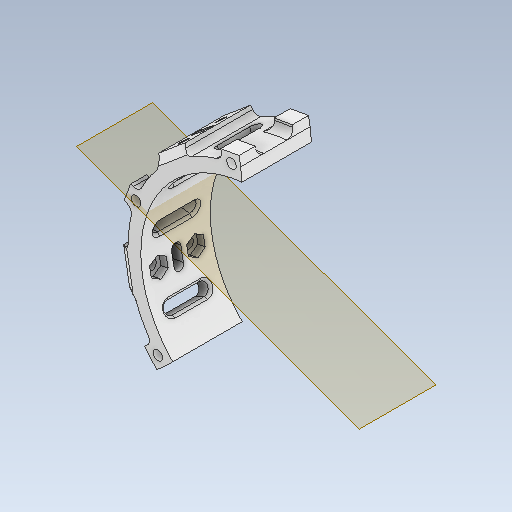
# Autodesk Inventor part: shell_3
Saved by Autodesk Inventor 2020 (Build 240168000, 168)
## iProperties
Created: 2020-07-11
Part Number: shell_3
Material: ABS Plastic
Document SubType Name: Modeling
Designer: psrobotics
Density: 1.06 g/cm^3
Appearance: Smooth - White
Author: psrobotics
Autodesk Inventor part; units mm, degrees
sketch "Sketch1" plane through (0, 0, 0) normal (0, 0, 1) x (1, 0, 0)
  line L0 (52.6477, -39.8597) -> (50.9677, -42.7938) projected
  line L1 (39.9879, -61.9696) -> (50.9677, -42.7938) projected
  circle A0 centre (0, 0) radius 5.9 projected
  circle A1 centre (0, 0) radius 45.5 projected
  circle A2 centre (0, 0) radius 48.5
  circle A3 centre (0, 0) radius 54
  line L2 (0, 0) -> (0, -54)
  line L3 (0, 0) -> (0, 54)
  line L4 (0, 0) -> (-18.4691, -50.7434)
  line L5 (-18.4691, -50.7434) -> (-18.4691, -50.7434)
  line L6 (-26.7139, -51.4672) -> (-12.6185, -56.5975)
  line L7 (-12.6185, -56.5975) -> (-10.2243, -50.0196)
  line L8 (-10.2243, -50.0196) -> (-24.3197, -44.8893)
  line L9 (-24.3197, -44.8893) -> (-26.7139, -51.4672)
  line L10 (-26.7139, -51.4672) -> (-10.2243, -50.0196) construction
  line L11 (-12.6185, -56.5975) -> (-24.3197, -44.8893) construction
  line L12 (-57.9288, -2.5987) -> (-55.3241, -17.3708)
  line L13 (-55.3241, -17.3708) -> (-48.4304, -16.1553)
  line L14 (-48.4304, -16.1553) -> (-51.0352, -1.3832)
  line L15 (-51.0352, -1.3832) -> (-57.9288, -2.5987)
  line L16 (-31.215, 48.8685) -> (-42.7056, 39.2266)
  line L17 (-42.7056, 39.2266) -> (-38.2061, 33.8643)
  line L18 (-38.2061, 33.8643) -> (-26.7154, 43.5062)
  line L19 (-26.7154, 43.5062) -> (-31.215, 48.8685)
  line L20 (26.7139, 51.4672) -> (12.6185, 56.5975)
  line L21 (12.6185, 56.5975) -> (10.2243, 50.0196)
  line L22 (10.2243, 50.0196) -> (24.3197, 44.8893)
  line L23 (24.3197, 44.8893) -> (26.7139, 51.4672)
  line L24 (-10.2243, -50.0196) -> (24.3197, 44.8893)
  point P0 (0, 0)
  point P1 (-9.3407, -47.592)
  point P2 (23.4361, 42.4617)
  point P3 (11.2424, 52.8167)
  point P4 (-28.6288, 45.7864)
  point P5 (-40.1194, 36.1446)
  point P6 (-53.9666, -1.9001)
  point P7 (-51.3618, -16.6722)
  point P8 (-25.3378, -47.6864)
  dimension "d0" = 97
  dimension "d1" = 108
  dimension "d2" = 54
  dimension "d3" = 20
  dimension "d4" = 0
  dimension "d5" = 15
  dimension "d6" = 7
  dimension "d9" = 180
  constraints: 46 end point, 2 centre point, 2 coincident, 2 midpoint, 2 parallel, 2 perpendicular, 2 point on circle, 2 vertical, 1 collinear, 25 other
  measures "d0" diameter of A2
  measures "d1" diameter of A3
  measures "d2" distance of L2.start L4.end
  measures "d3" angle of L2 L4
  measures "d4" distance of L4.end L5.end
  measures "d5" distance of L6.start L6.end
  measures "d6" distance of L7.end L6.end
extrude "Extrusion1" add sketch "Sketch1" against normal blind 30 contours L3 A3 L21 L22 L24 A2 | A2 L4 L8 L9 A3 L13 L14 L15 L17 L18 L19 L3 | A2 L24 L8 L4 | L8 L7 A3 L4 | L4 A3 L9 L8 | L22 L21 A3 L23 | L21 L20 L23 A3 | L19 L18 L17 A3 | A3 L17 L16 L19 | A3 L7 L6 L9 | L15 L14 L13 A3 | A3 L13 L12 L15
sketch "Sketch2" plane through (0, 0, -30) normal (0, 0, -1) x (-1, 0, 0)
  line L0 (57.9288, -2.5987) -> (53.9666, -1.9001) projected
  arc A0 (53.9666, -1.9001) -> (40.1194, 36.1446) centre (0, 0) ccw projected
  line L1 (40.1194, 36.1446) -> (42.7056, 39.2266) projected
  line L2 (42.7056, 39.2266) -> (31.215, 48.8685) projected
  line L3 (31.215, 48.8685) -> (28.6288, 45.7864) projected
  arc A1 (28.6288, 45.7864) -> (-11.2424, 52.8167) centre (0, 0) ccw projected
  line L4 (-11.2424, 52.8167) -> (-12.6185, 56.5975) projected
  line L5 (-12.6185, 56.5975) -> (-26.7139, 51.4672) projected
  line L6 (-26.7139, 51.4672) -> (-23.4361, 42.4617) projected
  arc A2 (9.3407, -47.592) -> (-23.4361, 42.4617) centre (0, 0) ccw projected
  line L7 (9.3407, -47.592) -> (12.6185, -56.5975) projected
  line L8 (12.6185, -56.5975) -> (26.7139, -51.4672) projected
  line L9 (26.7139, -51.4672) -> (25.3378, -47.6864) projected
  arc A3 (25.3378, -47.6864) -> (51.3618, -16.6722) centre (0, 0) ccw projected
  line L10 (51.3618, -16.6722) -> (55.3241, -17.3708) projected
  line L11 (55.3241, -17.3708) -> (57.9288, -2.5987) projected
  line L12 (0, 0) -> (-19.6662, 54.0323)
  line L13 (-26.7139, 51.4672) -> (-12.6185, 56.5975) projected
  line L14 (-16.588, 45.5751) -> (-23.6357, 43.0099)
  line L15 (-23.4361, 42.4617) -> (-26.7139, 51.4672) projected
  point P0 (0, 0)
  constraints: 4 end point, 2 perpendicular, 2 point on line, 1 midpoint, 1 point on circle
extrude "Extrusion2" cut sketch "Sketch2" against normal blind 50 contours A2 L6 L14
ref_plane "Work Plane1" through (7.0477, -2.5652, 0) normal (0.3420201, 0.9396926, 0) x (0.9396926, -0.3420201, 0)
mirror "Mirror1" about plane through (7.0477, -2.5652, 0) normal (0.3420201, 0.9396926, 0) of "Extrusion2"
sketch "Sketch3" plane through (0, 0, 0) normal (0, 0, 1) x (1, 0, 0)
  line L0 (-9.5403, -48.1402) -> (-16.588, -45.5751) projected
  arc A0 (16.588, 45.5751) -> (-16.588, -45.5751) centre (0, 0) ccw projected
  line L1 (16.588, 45.5751) -> (23.6357, 43.0099) projected
  line L2 (23.6357, 43.0099) -> (26.7139, 51.4672) projected
  line L3 (26.7139, 51.4672) -> (12.6185, 56.5975) projected
  line L4 (12.6185, 56.5975) -> (11.2424, 52.8167) projected
  arc A1 (11.2424, 52.8167) -> (-28.6288, 45.7864) centre (0, 0) ccw projected
  line L5 (-28.6288, 45.7864) -> (-31.215, 48.8685) projected
  line L6 (-31.215, 48.8685) -> (-42.7056, 39.2266) projected
  line L7 (-42.7056, 39.2266) -> (-40.1194, 36.1446) projected
  arc A2 (-40.1194, 36.1446) -> (-53.9666, -1.9001) centre (0, 0) ccw projected
  line L8 (-53.9666, -1.9001) -> (-57.9288, -2.5987) projected
  line L9 (-57.9288, -2.5987) -> (-55.3241, -17.3708) projected
  line L10 (-55.3241, -17.3708) -> (-51.3618, -16.6722) projected
  arc A3 (-51.3618, -16.6722) -> (-25.3378, -47.6864) centre (0, 0) ccw projected
  line L11 (-25.3378, -47.6864) -> (-26.7139, -51.4672) projected
  line L12 (-26.7139, -51.4672) -> (-12.6185, -56.5975) projected
  line L13 (-12.6185, -56.5975) -> (-9.5403, -48.1402) projected
  line L14 (-12.6185, -56.5975) -> (-26.7139, -51.4672) projected
  line L15 (-19.6662, -54.0323) -> (-56.6264, -9.9848)
  line L16 (-55.3241, -17.3708) -> (-57.9288, -2.5987) projected
  line L17 (0, 0) -> (-38.1463, -32.0085)
  line L18 (-38.1463, -32.0085) -> (-41.2105, -34.5797)
  line L19 (-41.7035, -40.215) -> (-46.8458, -34.0867)
  line L20 (-46.8458, -34.0867) -> (-40.7175, -28.9444)
  line L21 (-40.7175, -28.9444) -> (-35.5752, -35.0727)
  line L22 (-35.5752, -35.0727) -> (-41.7035, -40.215)
  line L23 (-41.7035, -40.215) -> (-40.7175, -28.9444) construction
  line L24 (-46.8458, -34.0867) -> (-35.5752, -35.0727) construction
  point P0 (0, 0)
  point P1 (-38.6816, -37.6793)
  point P2 (-43.8239, -31.551)
  dimension "d15" = 4
  dimension "d16" = 8
  dimension "d17" = 8
  constraints: 18 end point, 5 midpoint, 2 parallel, 2 perpendicular, 1 point on line
  measures "d15" distance of L17.end L18.end
  measures "d16" distance of L19.start L19.end
  measures "d17" distance of L19.end L20.end
extrude "Extrusion3" add sketch "Sketch3" against normal blind 7 contours L22 L19 L20 A3
pattern_circular "Circular Pattern1" count 3 over 120 about axis through (0, 0, 0) along (0, 0, -1) of "Extrusion3"
sketch "Sketch4" plane through (0, 0, 0) normal (0, 0, 1) x (1, 0, 0)
  line L0 (-9.5403, -48.1402) -> (-16.588, -45.5751) projected
  arc A0 (16.588, 45.5751) -> (-16.588, -45.5751) centre (0, 0) ccw projected
  line L1 (16.588, 45.5751) -> (23.6357, 43.0099) projected
  line L2 (23.6357, 43.0099) -> (26.7139, 51.4672) projected
  line L3 (26.7139, 51.4672) -> (12.6185, 56.5975) projected
  line L4 (12.6185, 56.5975) -> (11.2424, 52.8167) projected
  arc A1 (11.2424, 52.8167) -> (-5.412, 53.7281) centre (0, 0) ccw projected
  line L5 (-5.412, 53.7281) -> (-6.097, 57.613) projected
  line L6 (-6.097, 57.613) -> (-13.9755, 56.2238) projected
  line L7 (-13.9755, 56.2238) -> (-13.2905, 52.3389) projected
  arc A2 (-13.2905, 52.3389) -> (-28.6288, 45.7864) centre (0, 0) ccw projected
  line L8 (-28.6288, 45.7864) -> (-31.215, 48.8685) projected
  line L9 (-31.215, 48.8685) -> (-42.7056, 39.2266) projected
  line L10 (-42.7056, 39.2266) -> (-40.1194, 36.1446) projected
  arc A3 (-40.1194, 36.1446) -> (-49.2359, 22.1771) centre (0, 0) ccw projected
  line L11 (-49.2359, 22.1771) -> (-52.9428, 23.5263) projected
  line L12 (-52.9428, 23.5263) -> (-55.679, 16.0088) projected
  line L13 (-55.679, 16.0088) -> (-51.9721, 14.6596) projected
  arc A4 (-51.9721, 14.6596) -> (-53.9666, -1.9001) centre (0, 0) ccw projected
  line L14 (-53.9666, -1.9001) -> (-57.9288, -2.5987) projected
  line L15 (-57.9288, -2.5987) -> (-55.3241, -17.3708) projected
  line L16 (-55.3241, -17.3708) -> (-51.3618, -16.6722) projected
  arc A5 (-51.3618, -16.6722) -> (-43.8239, -31.551) centre (0, 0) ccw projected
  line L17 (-43.8239, -31.551) -> (-46.8458, -34.0867) projected
  line L18 (-46.8458, -34.0867) -> (-41.7035, -40.215) projected
  line L19 (-41.7035, -40.215) -> (-38.6816, -37.6793) projected
  arc A6 (-38.6816, -37.6793) -> (-25.3378, -47.6864) centre (0, 0) ccw projected
  line L20 (-25.3378, -47.6864) -> (-26.7139, -51.4672) projected
  line L21 (-26.7139, -51.4672) -> (-12.6185, -56.5975) projected
  line L22 (-12.6185, -56.5975) -> (-9.5403, -48.1402) projected
  line L23 (-44.2747, -37.1508) -> (-41.2105, -34.5797)
  line L24 (-46.8458, -34.0867) -> (-41.7035, -40.215) projected
  circle A7 centre (-41.2105, -34.5797) radius 2.05
  point P0 (0, 0)
  dimension "d23" = 4
  dimension "d24" = 4.1
  constraints: 2 end point, 1 centre point, 1 coincident, 1 midpoint, 1 perpendicular
  measures "d23" distance of L23.start L23.end
  measures "d24" diameter of A7
extrude "Extrusion4" cut sketch "Sketch4" against normal blind 5 contours A7
pattern_circular "Circular Pattern2" count 3 over 120 about axis through (0, 0, 0) along (0, 0, -1) of "Extrusion4"
ref_plane "Work Plane2" through (0, 0, -15) normal (0, 0, 1) x (1, 0, 0)
mirror "Mirror2" about plane through (0, 0, -15) normal (0, 0, 1) of "Extrusion3", "Circular Pattern1", "Extrusion4", "Circular Pattern2"
ref_plane "Work Plane3" through (-23.2937, -42.0702, -30) normal (-0.3420201, -0.9396926, 0) x (0.9396926, -0.3420201, 0)
sketch "Sketch5" plane through (-26.7139, -51.4672, -30) normal (-0.3420201, -0.9396926, 0) x (0.9396926, -0.3420201, 0)
  line L0 (0, 30) -> (15, 30) projected
  line L1 (0, 30) -> (0, 0) projected
  line L2 (15, 0) -> (0, 0) projected
  line L3 (15, 30) -> (15, 0) projected
  line L4 (15, 0) -> (0, 0) projected
  line L5 (7.5, 0) -> (7.5, 7)
  line L6 (7.5, 30) -> (7.5, 23)
  line L7 (7.5, 0) -> (7.5, 30) projected
  circle A0 centre (7.5, 23) radius 2.05
  circle A1 centre (7.5, 7) radius 2.05
  dimension "d31" = 7
  dimension "d32" = 7
  dimension "d33" = 4.1
  dimension "d34" = 4.1
  constraints: 4 end point, 2 centre point, 2 coincident, 1 midpoint, 1 point on line, 1 vertical
  measures "d31" distance of L5.start L5.end
  measures "d32" distance of L6.start L6.end
  measures "d33" diameter of A0
  measures "d34" diameter of A1
extrude "Extrusion5" cut sketch "Sketch5" against normal blind 15 contours A0 L7 L6 | L6 L7 A0 | A1 L7 L5 | L5 L7 A1
sketch "Sketch6" plane through (-23.2937, -42.0702, -30) normal (-0.3420201, -0.9396926, 0) x (0.9396926, -0.3420201, 0)
  circle A0 centre (7.5, 7) radius 2.05 projected
  circle A1 centre (7.5, 23) radius 2.05 projected
  line L0 (0, 30) -> (15, 30) projected
  line L1 (0, 30) -> (0, 0) projected
  line L2 (15, 0) -> (0, 0) projected
  line L3 (15, 30) -> (15, 0) projected
  line L4 (7.5, 23) -> (3.3, 23)
  line L5 (7.5, 23) -> (5.4, 19.3627)
  line L6 (7.5, 23) -> (9.6, 19.3627)
  line L7 (7.5, 23) -> (11.7, 23)
  line L8 (7.5, 23) -> (9.6, 26.6373)
  line L9 (7.5, 23) -> (5.4, 26.6373)
  line L10 (7.5, 7) -> (3.3, 7)
  line L11 (15, 0) -> (0, 0) projected
  line L12 (7.5, 7) -> (5.4, 3.3627)
  line L13 (7.5, 7) -> (9.6, 3.3627)
  line L14 (7.5, 7) -> (11.7, 7)
  line L15 (7.5, 7) -> (9.6, 10.6373)
  line L16 (7.5, 7) -> (5.4, 10.6373)
  line L17 (9.6, 26.6373) -> (11.7, 23)
  line L18 (11.7, 23) -> (9.6, 19.3627)
  line L19 (9.6, 19.3627) -> (5.4, 19.3627)
  line L20 (5.4, 19.3627) -> (3.3, 23)
  line L21 (3.3, 23) -> (5.4, 26.6373)
  line L22 (5.4, 26.6373) -> (9.6, 26.6373)
  line L23 (9.6, 10.6373) -> (5.4, 10.6373)
  line L24 (7.5, 9.05) -> (7.5, 20.95) projected
  line L25 (5.4, 10.6373) -> (3.3, 7)
  line L26 (3.3, 7) -> (5.4, 3.3627)
  line L27 (5.4, 3.3627) -> (9.6, 3.3627)
  line L28 (9.6, 3.3627) -> (11.7, 7)
  line L29 (11.7, 7) -> (9.6, 10.6373)
  point P0 (7.5, 30)
  dimension "d37" = 4.2
  dimension "d40" = 360
  dimension "d42" = 4.2
  dimension "d45" = 360
  constraints: 48 end point, 8 parallel, 4 coincident, 2 horizontal, 2 vertical alignment, 1 perpendicular, 34 other
  measures "d37" distance of L4.start L4.end
  measures "d42" distance of L10.start L10.end
extrude "Extrusion6" cut sketch "Sketch6" along normal blind 4.2 contours L14 L15 A0 | L14 L28 L13 A0 | A0 L13 L14 | A0 L15 L29 L14 | L15 L16 A0 | A0 L24 L23 L15 | L13 L27 L12 A0 | A0 L12 L13 | L12 A0 L10 | L10 A0 L16 | A0 L16 L23 L24 | L12 L26 L10 A0 | L10 L25 L16 A0 | L7 L8 A1 | L7 L18 L6 A1 | A1 L6 L7 | A1 L8 L17 L7 | L8 L9 A1 | A1 L9 L22 L8 | L6 L19 L24 A1 | A1 L5 L6 | L5 A1 L4 | L4 A1 L9 | A1 L4 L21 L9 | L24 L19 L5 A1 | A1 L5 L20 L4
pattern_circular "Circular Pattern3" count 4 over 180 about axis through (0, 0, 0) along (0, 0, -1) of "Extrusion5", "Extrusion6"
sketch "Sketch7" plane through (0, 0, 0) normal (0, 0, 1) x (1, 0, 0)
  circle A0 centre (-9.3417, 52.9792) radius 2.05 projected
  circle A1 centre (-50.5521, 18.3995) radius 2.05 projected
  circle A2 centre (-41.2105, -34.5797) radius 2.05 projected
  line L0 (-9.5403, -48.1402) -> (-16.588, -45.5751) projected
  arc A3 (16.588, 45.5751) -> (-16.588, -45.5751) centre (0, 0) ccw projected
  line L1 (16.588, 45.5751) -> (23.6357, 43.0099) projected
  line L2 (23.6357, 43.0099) -> (26.7139, 51.4672) projected
  line L3 (26.7139, 51.4672) -> (12.6185, 56.5975) projected
  line L4 (12.6185, 56.5975) -> (11.2424, 52.8167) projected
  arc A4 (11.2424, 52.8167) -> (-5.412, 53.7281) centre (0, 0) ccw projected
  line L5 (-5.412, 53.7281) -> (-6.097, 57.613) projected
  line L6 (-6.097, 57.613) -> (-13.9755, 56.2238) projected
  line L7 (-13.9755, 56.2238) -> (-13.2905, 52.3389) projected
  arc A5 (-13.2905, 52.3389) -> (-28.6288, 45.7864) centre (0, 0) ccw projected
  line L8 (-28.6288, 45.7864) -> (-31.215, 48.8685) projected
  line L9 (-31.215, 48.8685) -> (-42.7056, 39.2266) projected
  line L10 (-42.7056, 39.2266) -> (-40.1194, 36.1446) projected
  arc A6 (-40.1194, 36.1446) -> (-49.2359, 22.1771) centre (0, 0) ccw projected
  line L11 (-49.2359, 22.1771) -> (-52.9428, 23.5263) projected
  line L12 (-52.9428, 23.5263) -> (-55.679, 16.0088) projected
  line L13 (-55.679, 16.0088) -> (-51.9721, 14.6596) projected
  arc A7 (-51.9721, 14.6596) -> (-53.9666, -1.9001) centre (0, 0) ccw projected
  line L14 (-53.9666, -1.9001) -> (-57.9288, -2.5987) projected
  line L15 (-57.9288, -2.5987) -> (-55.3241, -17.3708) projected
  line L16 (-55.3241, -17.3708) -> (-51.3618, -16.6722) projected
  arc A8 (-51.3618, -16.6722) -> (-43.8239, -31.551) centre (0, 0) ccw projected
  line L17 (-43.8239, -31.551) -> (-46.8458, -34.0867) projected
  line L18 (-46.8458, -34.0867) -> (-41.7035, -40.215) projected
  line L19 (-41.7035, -40.215) -> (-38.6816, -37.6793) projected
  arc A9 (-38.6816, -37.6793) -> (-25.3378, -47.6864) centre (0, 0) ccw projected
  line L20 (-25.3378, -47.6864) -> (-26.7139, -51.4672) projected
  line L21 (-26.7139, -51.4672) -> (-12.6185, -56.5975) projected
  line L22 (-12.6185, -56.5975) -> (-9.5403, -48.1402) projected
  line L23 (-38.6816, -37.6793) -> (-41.7035, -40.215) projected
  line L24 (0, 0) -> (-38.6816, -37.6793)
  line L25 (0, 0) -> (-5.412, 53.7281)
  point P0 (0, 0)
  point P1 (-4.8608, 48.2558)
  point P2 (-34.7418, -33.8416)
  constraints: 4 end point
extrude "Extrusion7" cut sketch "Sketch7" against normal up to surface (30 mm away) contours L22 L21 L20 A9 L24 A3 L0 | L25 A4 L4 L3 L2 L1 A3
sketch "Sketch8" plane through (-31.215, 48.8685, 0) normal (-0.6427876, 0.7660444, 0) x (0.7660444, 0.6427876, 0)
  line L0 (-5.4, 10.6373) -> (-9.6, 10.6373) projected
  line L1 (-9.6, 19.3627) -> (-5.4, 19.3627) projected
  line L2 (-7.5, 10.6373) -> (-7.5, 19.3627)
  line L3 (-4.5, 15) -> (-10.5, 15) construction
  line L4 (-4.5, 17) -> (-10.5, 17)
  line L5 (-10.5, 13) -> (-4.5, 13)
  arc A0 (-4.5, 13) -> (-4.5, 17) centre (-4.5, 15) ccw
  arc A1 (-10.5, 17) -> (-10.5, 13) centre (-10.5, 15) ccw
  point P0 (-7.5, 0)
  point P1 (-7.5, 15)
  dimension "d54" = 3
  dimension "d55" = 4
  constraints: 10 end point, 4 midpoint, 4 point on circle, 4 tangent, 2 centre point, 1 parallel, 1 perpendicular
  measures "d54" distance of point (-7.5, 15) L3.end
  measures "d55" diameter of A1
extrude "Extrusion8" cut sketch "Sketch8" against normal blind 10
pattern_circular "Circular Pattern4" count 2 over 60 about axis through (0, 0, 0) along (0, 0, 1) of "Extrusion8"
fillet "Fillet1" radius 3 14 edges at (-13.2905, 52.3389, -3.5) (-13.2905, 52.3389, -26.5) (-49.2359, 22.1771, -26.5) (-49.2359, 22.1771, -3.5) (-51.9721, 14.6596, -3.5) (-51.9721, 14.6596, -26.5) (-43.8239, -31.551, -3.5) (-43.8239, -31.551, -26.5) (-41.3664, -34.7105, -23) (-41.3664, -34.7105, -7) (-50.7434, 18.4691, -7) (-50.7434, 18.4691, -23) (-9.377, 53.1796, -23) (-9.377, 53.1796, -7)
fillet "Fillet2" radius 3 4 edges at (-28.6288, 45.7864, -15) (-40.1194, 36.1446, -15) (-53.9666, -1.9001, -15) (-51.3618, -16.6722, -15)
chamfer "Chamfer1" distance 2 angle 60 1 edges at (-36.9603, 44.0476, 0) measured on face at (-36.9603, 44.0476, -0.5)
chamfer "Chamfer2" distance 2 angle 60 1 edges at (-56.6264, -9.9848, 0) measured on face at (-56.6264, -9.9848, -0.5)
ref_plane "Work Plane4" through (-31.215, 48.8685, 0) normal (0.3924314, -0.9197813, 0) x (0, 0, -1)
sketch "Sketch9" plane through (-31.215, 48.8685, 0) normal (0.3924314, -0.9197813, 0) x (0, 0, -1)
  line L0 (0, 3.6274) -> (30, 3.6274) projected
  line L1 (0, 15.2264) -> (0, 3.6274) projected
  line L2 (10, 15.2264) -> (0, 15.2264) projected
  line L3 (10, 25.6401) -> (10, 15.2264) projected
  line L4 (10, 25.6401) -> (20, 25.6401) projected
  line L5 (20, 15.2264) -> (20, 25.6401) projected
  line L6 (30, 15.2264) -> (20, 15.2264) projected
  line L7 (30, 3.6274) -> (30, 15.2264) projected
  line L8 (30, 15.2264) -> (0, 3.6274)
  line L9 (30, 3.6274) -> (0, 15.2264)
  line L10 (8, 9.4269) -> (22, 9.4269) construction
  line L11 (8, 6.9269) -> (22, 6.9269)
  line L12 (22, 11.9269) -> (8, 11.9269)
  arc A0 (8, 11.9269) -> (8, 6.9269) centre (8, 9.4269) ccw
  arc A1 (22, 6.9269) -> (22, 11.9269) centre (22, 9.4269) ccw
  point P0 (0, 9.5334)
  point P1 (15, 9.4269)
  dimension "d69" = 7
  dimension "d70" = 5
  constraints: 12 end point, 4 point on circle, 4 tangent, 2 centre point, 2 midpoint, 1 horizontal, 1 parallel
  measures "d69" distance of point (15, 9.427) L10.end
  measures "d70" diameter of A1
extrude "Extrusion9" cut sketch "Sketch9" along normal blind 10 contours L11 A0 L12 L9 L8 | L8 L9 L11 | L9 L8 L12 A1 L11 | L12 L8 L9
ref_plane "Work Plane5" through (-42.7056, 39.2266, 0) normal (-0.8376627, 0.5461878, 0) x (0, 0, -1)
sketch "Sketch10" plane through (-42.7056, 39.2266, 0) normal (-0.8376627, 0.5461878, 0) x (0, 0, -1)
  line L0 (0, 38.5402) -> (30, 38.5402) projected
  line L1 (0, 28.1441) -> (0, 38.5402) projected
  line L2 (10, 28.1441) -> (0, 28.1441) projected
  line L3 (10, 15.2264) -> (10, 28.1441) projected
  line L4 (0, 15.2264) -> (10, 15.2264) projected
  line L5 (0, 3.6274) -> (0, 15.2264) projected
  line L6 (30, 3.6274) -> (0, 3.6274) projected
  line L7 (30, 15.2264) -> (30, 3.6274) projected
  line L8 (20, 15.2264) -> (30, 15.2264) projected
  line L9 (20, 28.1441) -> (20, 15.2264) projected
  line L10 (30, 28.1441) -> (20, 28.1441) projected
  line L11 (30, 38.5402) -> (30, 28.1441) projected
  ellipse E0 centre (1.1481, 3.2993) end of major axis (0.4413, 6.2757) minor radius 1.6252 (0, 1.728) -> (1.1481, 0.4288) ccw projected
  line L12 (1.1481, 0.4288) -> (30, 0.4288) projected
  line L13 (30, 0.4288) -> (30, 3.6274) projected
  line L14 (30, 3.6274) -> (0, 3.6274) projected
  line L15 (0, 3.6274) -> (0, 1.728) projected
  line L16 (30, 15.2264) -> (0, 3.6274)
  line L17 (0, 15.2264) -> (30, 3.6274)
  line L18 (8, 9.4269) -> (22, 9.4269) construction
  line L19 (8, 6.9269) -> (22, 6.9269)
  line L20 (22, 11.9269) -> (8, 11.9269)
  arc A0 (8, 11.9269) -> (8, 6.9269) centre (8, 9.4269) ccw
  arc A1 (22, 6.9269) -> (22, 11.9269) centre (22, 9.4269) ccw
  point P0 (0, 9.5334)
  point P1 (15, 9.4269)
  dimension "d73" = 7
  dimension "d74" = 5
  constraints: 12 end point, 4 point on circle, 4 tangent, 2 centre point, 2 midpoint, 1 horizontal, 1 parallel, 1 other
  measures "d73" distance of point (15, 9.427) L18.end
  measures "d74" diameter of A1
extrude "Extrusion10" cut sketch "Sketch10" against normal blind 10 contours L20 L16 L17 | L17 L16 L19 A0 L20 | L20 A1 L19 L17 L16 | L16 L17 L19
mirror "Mirror3" about plane through (7.0477, -2.5652, 0) normal (0.3420201, 0.9396926, 0) of "Extrusion9", "Extrusion10"
chamfer "Chamfer3" distance 1 angle 45 16 edges at (-44.3709, -19.5824, -15) (-43.4708, -21.5068, -24.4715) (-42.119, -24.0466, -15) (-43.3216, -21.8058, -5.5004) (-48.1162, 6.0894, -5.5285) (-47.8034, 8.1908, -15) (-48.1569, 5.7591, -24.4996) (-48.3926, 3.2257, -15) (-40.5451, 26.6147, -5.5004) (-39.1443, 28.6352, -15) (-40.3608, 26.8934, -24.4715) (-41.8844, 24.4529, -15) (-18.7846, 44.7145, -5.5285) (-16.8082, 45.4943, -15) (-19.0909, 44.5846, -24.4996) (-21.4028, 43.5221, -15)
body "Solid1"
